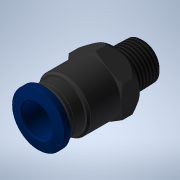
# Autodesk Inventor part: 153004 QS-1/8-8
Saved by Autodesk Inventor 2021 (Build 250183000, 183)
## iProperties
Created: 2025-06-05
Part Number: 153004 QS-1/8-8
Material: Generic
Catalog Web Link: www.cadenas.de
Description: QS-R-Push-in fitting
Vendor: FESTO
Document SubType Name: Modeling
Designer: psAdmin
Manufacturer: FESTO
Mass: 14 g
Surface Area: 21.0893 cm^2
Volume: 2.18489 cm^3
Density: 1 g/cm^3
Appearance: PSOLRGB-175-175-175
Category: PARTsolutions
Company: FESTO
Title: 153004 QS-1/8-8
Author: Cadenas PARTsolutions
Comments: Push-in fitting
PSOL_IDENT_0: {$CADENAS_DATA/23d-libs/festo/parts/q/qs/qs_r.prj},168 {VTYP=3D},{NB=153004 QS-1/8-8},{LINA=153004 Q
PSOL_IDENT_1: S-1/8-8},{NN=QS-R},{DATE=02.05.2025 12:35:03},{GEOMDATE=01.04.2025 10:00:38},{VERSION=},{LINEID=30},
PSOL_IDENT_2: {WBVAR=},{WBNUMERIC=}  {NB=153004 QS-1/8-8},{LINA=153004 QS-1/8-8},{KT=DUMMY},{TNR=153004},{TYP=QS-1
PSOL_IDENT_3: /8-8},{D1=R1/8},{NENN=6.000},{D2=8.000},{D5=13.700},{L2=8.000},{L1=27.900},{L3=23.900},{T=18.200},{S
PSOL_IDENT_4: W=14.000},{CNSMASSEXACT=0.0140},{Z=13.800},{VERS=1.000},{L6=3.800},{D5L=8.300},{D1N=9.728},{ZOLL=1/8
PSOL_IDENT_5: },{SH38=1.000},{DNC=0},{GTIN=4052568031145},{REACH=Ja},{REACHSVHC=Ja},{REACHHAZSUBS=7439-92-1},{REAC
PSOL_IDENT_6: HSCIP=3732228b-b396-49b9-8f0d-ee75d35d3f40},{REACHVALDATE=05.03.2025}
NB: 153004 QS-1/8-8
NN: QS-R
NT: Push-in fitting
NBSYN: $TNR. $TYP.
LINA: 153004 QS-1/8-8
CATALOG: Festo
TNR: 153004
TYP: QS-1/8-8
D1: R1/8
NENN: 6
D2: 8
D5: 13.7
L2: 8
L1: 27.9
L3: 23.9
T: 18.2
SW: 14
CNSMASSEXACT: 0.014
GTIN: 4052568031145
REACH: Yes
REACHSVHC: Yes
REACHHAZSUBS: 7439-92-1
REACHVALDATE: 05.03.2025
SUPPLIER: FESTO
ARTICLENO: 153004 QS-1/8-8
BOMINFO: 153004 QS-1/8-8
CREATOR: CADENAS GmbH
Autodesk Inventor part; units mm, degrees
sketch "Sketch_2" plane through (0, 0, 0) normal (1, 0, 0) x (0, 1, 0)
  line L0 (0, 0) -> (0, 19.9)
  line L1 (0, 19.9) -> (4.3, 19.9)
  line L2 (4.3, 19.9) -> (6.7347, 19.4707)
  arc A0 (6.9, 19.2737) -> (6.7347, 19.4707) centre (6.7, 19.2737) ccw
  line L3 (6.9, 19.2737) -> (6.9, 17.9)
  line L4 (6.9, 17.9) -> (4.7, 17.9)
  arc A1 (4.7, 17.9) -> (4.4, 17.6) centre (4.7, 17.6) ccw
  line L5 (4.4, 17.6) -> (4.4, 16.9)
  line L6 (4.4, 16.9) -> (5.7, 16.9)
  line L7 (5.7, 16.9) -> (5.9, 16.7)
  line L8 (5.9, 16.7) -> (5.9, 16)
  line L9 (5.9, 16) -> (5.8, 15.9)
  line L10 (5.8, 15.9) -> (5.9, 15.8)
  line L11 (5.9, 15.8) -> (5.9, 13.1)
  line L12 (5.9, 13.1) -> (8.4, 13.1)
  line L13 (8.4, 13.1) -> (8.4, 2.4249)
  line L14 (8.4, 2.4249) -> (7, 0)
  line L15 (7, 0) -> (0, 0)
  line L16 (0, 0) -> (0, 19.9)
  constraints: 34 end point, 4 point on circle, 2 centre point
revolve "Revolution1" add sketch "Sketch_2" angle 360 about axis through (0, 0, 0) along (0, 0, -1)
sketch "Sketch_3" plane through (0, 0, 0) normal (0, 0, 1) x (1, 0, 0)
  line L0 (-14, -14) -> (14, -14)
  line L1 (14, -14) -> (14, 14)
  line L2 (14, 14) -> (-14, 14)
  line L3 (-14, 14) -> (-14, -14)
  line L4 (-7, -4.0415) -> (0, -8.0829)
  line L5 (0, -8.0829) -> (7, -4.0415)
  line L6 (7, -4.0415) -> (7, 4.0415)
  line L7 (7, 4.0415) -> (0, 8.0829)
  line L8 (0, 8.0829) -> (-7, 4.0415)
  line L9 (-7, 4.0415) -> (-7, -4.0415)
  constraints: 20 end point
extrude "Extrusion1" cut sketch "Sketch_3" along normal blind 13.2
sketch "Sketch_4" plane through (0, 0, 0) normal (1, 0, 0) x (0, 1, 0)
  line L0 (0, -50) -> (0, 50)
  line L1 (6.35, 13.1) -> (6.6964, 12.5)
  line L2 (6.6964, 12.5) -> (6.85, 12.5)
  line L3 (6.85, 12.5) -> (6.85, 4.8)
  line L4 (6.85, 4.8) -> (16.85, 2.1205)
  line L5 (16.85, 2.1205) -> (16.85, 13.1)
  line L6 (16.85, 13.1) -> (6.35, 13.1)
  constraints: 14 end point
revolve "Revolution2" cut sketch "Sketch_4" angle 360 about axis through (0, 0, -50) along (0, 0, -1)
sketch "Sketch_6" plane through (0, 0, 0) normal (1, 0, 0) x (0, 1, 0)
  line L0 (0, -8) -> (0, 0)
  line L1 (0, 0) -> (4.9889, 0)
  line L2 (4.9889, 0) -> (4.7578, -7.4003)
  line L3 (4.7578, -7.4003) -> (4.1581, -8)
  line L4 (4.1581, -8) -> (0, -8)
  line L5 (0, -8) -> (0, 0)
  constraints: 12 end point
revolve "Revolution3" add sketch "Sketch_6" angle 360 about axis through (0, 0, -8) along (0, 0, -1)
thread "Thread1" size "R 1/8" standard "ISO Taper" length 6.4034
sketch "Sketch_5" plane through (0, 0, 0) normal (1, 0, 0) x (0, 1, 0)
  line L0 (0, -8) -> (0, 19.9)
  line L1 (0, 19.9) -> (4.3, 19.9)
  arc A0 (4.3, 19.9) -> (4, 19.6) centre (4.3, 19.6) ccw
  line L2 (4, 19.6) -> (4, 1.7)
  line L3 (4, 1.7) -> (3, 1.7)
  line L4 (3, 1.7) -> (3, -4.0389)
  line L5 (3, -4.0389) -> (2.7794, -4)
  line L6 (2.7794, -4) -> (2.7794, -7.5)
  line L7 (2.7794, -7.5) -> (3.2794, -8)
  line L8 (3.2794, -8) -> (0, -8)
  line L9 (0, -8) -> (0, 19.9)
  constraints: 20 end point, 2 point on circle, 1 centre point
revolve "Revolution4" cut sketch "Sketch_5" angle 360 about axis through (0, 0, -8) along (0, 0, -1)
ref_plane "ANBAU_XY" through (0, 0, -4) normal (0, 0, 1) x (1, 0, 0)
ref_plane "ANBAU_YZ" through (0, 0, -4) normal (1, 0, 0) x (0, 1, 0)
ref_plane "ANBAU_ZX" through (0, 0, -4) normal (0, 1, 0) x (0, 0, 1)
ref_plane "ANBAU_FDT3D_XY" through (0, 0, -4) normal (0, 0, -1) x (1, 0, 0)
ref_plane "ANBAU_FDT3D_YZ" through (0, 0, -4) normal (1, 0, 0) x (0, -1, 0)
ref_plane "ANBAU_FDT3D_ZX" through (0, 0, -4) normal (0, -1, 0) x (0, 0, -1)
ref_plane "ANBAU_STD_XY" through (0, 0, -4) normal (0, 0, 1) x (1, 0, 0)
ref_plane "ANBAU_STD_YZ" through (0, 0, -4) normal (1, 0, 0) x (0, 1, 0)
ref_plane "ANBAU_STD_ZX" through (0, 0, -4) normal (0, 1, 0) x (0, 0, 1)
ref_plane "DROSSEL_XY" through (0, 0, -4) normal (0, 0, -1) x (1, 0, 0)
ref_plane "DROSSEL_YZ" through (0, 0, -4) normal (1, 0, 0) x (0, -1, 0)
ref_plane "DROSSEL_ZX" through (0, 0, -4) normal (0, -1, 0) x (0, 0, -1)
ref_plane "FDT_SCHLAUCH_XY" through (0, 0, 1.7) normal (0, 0, 1) x (1, 0, 0)
ref_plane "FDT_SCHLAUCH_YZ" through (0, 0, 1.7) normal (1, 0, 0) x (0, 1, 0)
ref_plane "FDT_SCHLAUCH_ZX" through (0, 0, 1.7) normal (0, 1, 0) x (0, 0, 1)
ref_plane "TO_CAP_XY" through (0, 0, 19.9) normal (0, 0, 1) x (1, 0, 0)
ref_plane "TO_CAP_YZ" through (0, 0, 19.9) normal (1, 0, 0) x (0, 1, 0)
ref_plane "TO_CAP_ZX" through (0, 0, 19.9) normal (0, 1, 0) x (0, 0, 1)
body "Solid1"
